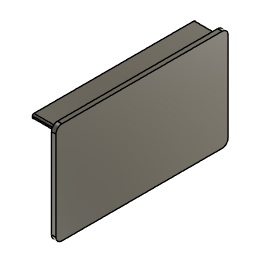
tapa+arduino (Autodesk Fusion 360 design; units mm, degrees)
Autodesk Fusion 360 part; units mm, degrees
sketch "Boceto1" plane through (0, 0, 0) normal (1, 0, 0) x (0, 1, 0)
  line L0 (-54.5, 54) -> (54.5, 54)
  line L1 (54.5, 54) -> (54.5, 0)
  line L2 (54.5, 0) -> (-54.5, 0)
  line L3 (-54.5, 0) -> (-54.5, 54)
  dimension "d4" = 54
  dimension "d5" = 109
  constraint horizontal L0
  constraint vertical L1
  constraint horizontal L2
  constraint vertical L3
  constraint midpoint origin L2
  measures "d4" distance of L0.start L2.end
  measures "d5" distance of L0.start L0.end
extrude "Extruir1" add sketch "Boceto1" along normal blind 14 makes body 1
sketch "Boceto2" plane through (0, 0, 0) normal (-1, 0, 0) x (0, -1, 0)
  line L0 (-54.5, 0) -> (54.5, 0)
  line L1 (54.5, 0) -> (54.5, 54)
  line L2 (54.5, 54) -> (-54.5, 54)
  line L3 (-54.5, 54) -> (-54.5, 0)
  line L4 (-58, -3.5) -> (-58, 64.2)
  line L5 (-58, 64.2) -> (-51.5, 64.2)
  line L6 (-51.5, 64.2) -> (-51.5, 61.2)
  line L7 (-51.5, 61.2) -> (-55, 61.2)
  line L8 (-55, 61.2) -> (-55, 57.5)
  line L9 (-55, 57.5) -> (-51.5, 57.5)
  line L10 (-51.5, 57.5) -> (-51.5, 54.5)
  line L11 (-51.5, 54.5) -> (-55, 54.5)
  line L12 (-55, 54.5) -> (-55, -0.5)
  line L13 (-55, -0.5) -> (0, -0.5)
  line L14 (-58, -3.5) -> (0, -3.5)
  line L15 (0, 2.5) -> (0, 20)
  line L16 (58, -3.5) -> (0, -3.5)
  line L17 (55, -0.5) -> (0, -0.5)
  line L18 (55, 54.5) -> (55, -0.5)
  line L19 (58, -3.5) -> (58, 64.2)
  line L20 (51.5, 54.5) -> (55, 54.5)
  line L21 (51.5, 57.5) -> (51.5, 54.5)
  line L22 (55, 57.5) -> (51.5, 57.5)
  line L23 (55, 61.2) -> (55, 57.5)
  line L24 (51.5, 61.2) -> (55, 61.2)
  line L25 (51.5, 64.2) -> (51.5, 61.2)
  line L26 (58, 64.2) -> (51.5, 64.2)
  line L27 (51.5, 64.2) -> (-51.5, 64.2)
  dimension "d10" = 0.5
  dimension "d11" = 3.7
  dimension "d12" = 3.5
  dimension "d13" = 0.5
  dimension "d14" = 0.5
  dimension "d15" = 3
  dimension "d16" = 3
  dimension "d17" = 3
  dimension "d18" = 3
  constraint vertical L8
  constraint perpendicular L8 L9
  constraint perpendicular L9 L10
  constraint vertical origin L13.end
  constraint vertical L13.end L14.end
  constraint horizontal L11
  constraint horizontal L7
  constraint horizontal L5
  constraint vertical L6
  constraint vertical L4
  constraint vertical L12
  constraint horizontal L14
  constraint horizontal L13
  constraint coincident L8 L11.end
  constraint coincident L6 L9.end
  constraint symmetric L4.start L15 L16.start
  constraint symmetric L4.end L15 L19.end
  constraint symmetric L5.end L15 L25.start
  constraint symmetric L6.end L15 L24.start
  constraint symmetric L7.end L15 L23.start
  constraint symmetric L8.end L15 L22.start
  constraint symmetric L9.end L15 L21.start
  constraint symmetric L10.end L15 L20.start
  constraint symmetric L11.end L15 L18.start
  constraint symmetric L12.end L15 L17.start
  constraint symmetric L13.end L15 L17.end
  constraint symmetric L14.end L15 L16.end
  measures "d10" distance of origin L13.end
  measures "d11" distance of L7.end L8.end
  measures "d12" distance of L6.end L7.end
  measures "d13" distance of L3 L12
  measures "d14" distance of L2 L11
  measures "d15" distance of L4 L12
  measures "d16" distance of L13 L14
  measures "d17" distance of L5.end L6.end
  measures "d18" distance of L9.end L10.end
extrude "Extruir2" add sketch "Boceto2" along normal blind 0 and the other way blind 16 separate body contours L4 L5 L6 L7 L8 L9 L10 L11 L12 L13 L14 L16 L17 L18 L19 L20 L21 L22 L23 L24 L25 L26 makes body 2
extrude "Extruir3" add sketch "Boceto2" along normal blind 3 contours L0 L1 L2 L3 | L4 L5 L6 L7 L8 L9 L10 L11 L12 L13 L14 L16 L17 L18 L19 L20 L21 L22 L23 L24 L25 L26 | L6 L7 L8 L9 L10 L11 L12 L13 L17 L18 L20 L21 L22 L23 L24 L25 L27 bodies 2
fillet "Empalme1" radius 4 4 edges at (6.5, 58, 64.2) (6.5, 58, -3.5) (6.5, -58, 64.2) (6.5, -58, -3.5) on bodies 2
fillet "Empalme2" radius 0.5 8 edges at (8, 51.5, 64.2) (8, 51.5, 54.5) (8, 51.5, 57.5) (8, 51.5, 61.2) (8, -51.5, 54.5) (8, -51.5, 61.2) (8, -51.5, 64.2) (8, -51.5, 57.5) on bodies 2
sketch "Boceto3" plane through (0, 0, 0) normal (0, 1, 0) x (1, 0, 0)
  line L0 (19.3, -64.2) -> (16.3, -64.2)
  line L1 (16.3, -64.2) -> (16.3, 3.5)
  line L2 (16.3, 3.5) -> (19.3, 3.5)
  line L3 (19.3, 3.5) -> (19.3, -64.2)
  line L4 (16.3, -60.85) -> (0.6, -60.85)
  line L5 (0.6, -60.85) -> (0.6, -57.85)
  line L6 (0.6, -57.85) -> (16.3, -57.85)
  line L7 (16.3, -57.85) -> (16.3, -60.85)
  line L8 (0, -61.2) -> (0, -57.5)
  line L9 (16, -61.2) -> (0, -61.2)
  point P0 (16, 3.5)
  point P1 (16, -64.2)
  dimension "d29" = 3
  dimension "d30" = 0.6
  dimension "d31" = 0.35
  dimension "d32" = 0.3
  dimension "d33" = 3
  constraint horizontal L0
  constraint vertical L1
  constraint horizontal L2
  constraint vertical L3
  constraint horizontal L4
  constraint vertical L5
  constraint horizontal L6
  constraint vertical L7
  constraint coincident L1 L4.start
  constraint coincident L2 P0
  constraint coincident L0 P1
  measures "d29" distance of L4.end L5.end
  measures "d30" distance of L5 L8
  measures "d31" distance of L4 L9
  measures "d32" distance of L1 P1
  measures "d33" distance of L0.start L0.end
extrude "Extruir4" add sketch "Boceto3" along normal mid plane 109 separate body contours L1 L4 L5 L6 L7 makes body 3
extrude "Extruir5" add sketch "Boceto3" along normal mid plane 115 contours L0 L1 L2 L3 L7 bodies 3
fillet "Empalme3" radius 4 4 edges at (17.8, 57.5, 64.2) (17.8, -57.5, 64.2) (17.8, -57.5, -3.5) (17.8, 57.5, -3.5) on bodies 3
fillet "Empalme4" radius 1.5 4 edges at (16.3, 0, 57.85) (16.3, -54.5, 59.35) (16.3, 0, 60.85) (16.3, 54.5, 59.35) on bodies 3
fillet "Empalme5" radius 1 8 edges at (7.7, 54.5, 60.85) (15.8607, 54.9393, 61.2893) (15.8607, 54.9393, 57.4107) (7.7, 54.5, 57.85) (15.8607, -54.9393, 61.2893) (7.7, -54.5, 60.85) (7.7, -54.5, 57.85) (15.8607, -54.9393, 57.4107) on bodies 3
hidden bodies 1 2
equation "largo = 14 mm"
equation "ancho = 109 mm"
equation "alto = 54 mm"
equation "d4 = alto"
equation "d5 = ancho"
equation "d6 = largo"
equation "d21 = largo + 2 mm"
equation "d36 = ancho"
equation "d38 = ancho + 6 mm"
